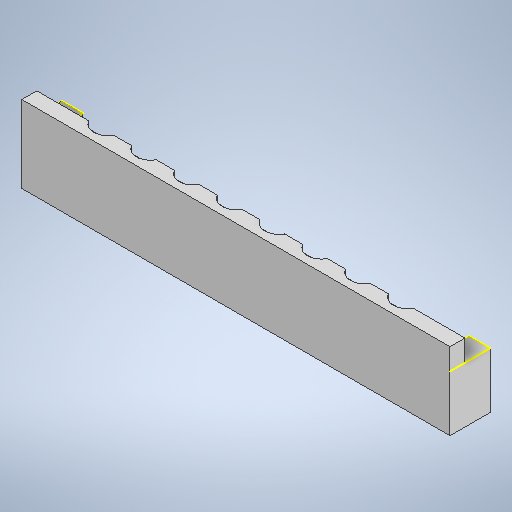
# Autodesk Inventor part: plate holder
Saved by Autodesk Inventor 2025.1 (Build 291241020, 241B)
## iProperties
Created: 2024-12-05
Part Number: plate holder
Material: Generic
Document SubType Name: Modeling
Designer: Hunter Mathis
Density: 1 g/cm^3
Appearance: Default
Author: Hunter Mathis
Autodesk Inventor part; units mm, degrees
ref_plane "YZ Plane" through (0, 0, 0) normal (1, 0, 0) x (0, 1, 0)
ref_plane "XZ Plane" through (0, 0, 0) normal (0, 1, 0) x (-1, 0, 0)
ref_plane "XY Plane" through (0, 0, 0) normal (0, 0, 1) x (1, 0, 0)
sketch "Sketch1" plane through (0, 0, 0) normal (0, 1, 0) x (-1, 0, 0)
  line L0 (63.5, -2.2225) -> (-63.5, -2.2225)
  line L1 (-63.5, -2.2225) -> (-63.5, 2.2225)
  line L2 (-63.5, 2.2225) -> (63.5, 2.2225)
  line L3 (63.5, 2.2225) -> (63.5, -2.2225)
  line L4 (63.5, -2.2225) -> (-63.5, 2.2225) construction
  line L5 (-63.5, -2.2225) -> (63.5, 2.2225) construction
  point P0 (0, 0)
  dimension "d0" = 127
  dimension "d1" = 4.445
  constraints: 12 end point, 2 midpoint, 2 parallel, 1 horizontal, 1 perpendicular
  measures "d0" distance of L1.end L2.end
  measures "d1" distance of L0.end L1.end
extrude "Extrusion1" add sketch "Sketch1" along normal blind 31.75
sketch "Sketch2" plane through (63.5, 0, -2.2225) normal (0, 0, -1) x (-1, 0, 0)
  line L0 (127, 0) -> (0, 0) projected
  line L1 (0, 0) -> (127, 0)
  line L2 (127, 0) -> (127, 25.4116)
  line L3 (127, 25.4116) -> (0, 25.4116)
  line L4 (0, 25.4116) -> (0, 0)
  point P0 (63.5, 0)
  constraints: 8 end point, 3 equal length, 1 perpendicular
extrude "Extrusion2" add sketch "Sketch2" along normal blind 7.4676
sketch "Sketch3" plane through (-63.5, 25.4116, -2.2225) normal (0, 1, 0) x (1, 0, 0)
  point P0 (63.5, -2.2225)
sketch "Sketch4" plane through (63.5, 0, -9.6901) normal (0, 0, -1) x (-1, 0, 0)
  line L0 (0, 25.4116) -> (0, 0) projected
  line L1 (6.223, 12.7058) -> (6.223, 25.4116)
  line L2 (0, 25.4116) -> (6.223, 25.4116)
  line L3 (0, 25.4116) -> (0, 12.7058)
  line L4 (0, 12.7058) -> (0, 3.1808)
  line L5 (0, 0) -> (0, 31.75) projected
  line L6 (0, 3.1808) -> (6.223, 3.1808)
  line L7 (6.223, 3.1808) -> (6.223, 12.7058)
  line L8 (0, 25.4116) -> (127, 25.4116) projected
  line L9 (127, 0) -> (127, 25.4116) projected
  line L10 (120.777, 12.7058) -> (120.777, 25.4116)
  line L11 (6.223, 25.4116) -> (120.777, 25.4116)
  line L12 (120.777, 12.7058) -> (120.777, 3.1808)
  line L13 (120.777, 3.1808) -> (127, 3.1808)
  line L14 (127, 3.1808) -> (127, 25.4116)
  line L15 (127, 0) -> (127, 31.75) projected
  line L16 (6.223, 3.1808) -> (120.777, 3.1808)
  line L17 (6.223, 3.1808) -> (6.223, 22.2308)
  line L18 (120.777, 22.2308) -> (6.223, 22.2308)
  line L19 (120.777, 22.2308) -> (120.777, 3.1808)
  line L20 (6.223, 3.1808) -> (120.777, 3.1808)
  point P0 (63.5, 0)
  point P1 (6.223, 22.2308)
  dimension "d6" = 6.223
  dimension "d7" = 9.525
  dimension "d13" = 6.223
  dimension "d14" = 19.05
  constraints: 32 end point, 5 collinear, 5 point on line, 4 perpendicular, 1 horizontal, 1 midpoint, 1 parallel, 1 vertical
  measures "d6" distance of L3.end L1.start
  measures "d7" distance of L3.end L4.end
  measures "d13" distance of L12.end L13.end
  measures "d14" distance between parallel lines of L18 L16
extrude "Extrusion3" cut sketch "Sketch4" against normal blind 4.699 contours L8 L10 L18 L1 | L18 L10 L12 L16 L7 L1
extrude "Extrusion4" add sketch "Sketch4" against normal blind 1.143 contours L18 L10 L12 L16 L7 L1
sketch "Sketch5" plane through (-63.5, 25.4116, -2.2225) normal (0, 1, 0) x (1, 0, 0)
  line L0 (127, -4.445) -> (127, 7.4676) projected
  line L1 (120.777, 7.4676) -> (120.777, 2.7686) projected
  line L2 (6.223, 2.7686) -> (6.223, 7.4676) projected
  line L3 (0, 7.4676) -> (6.223, 7.4676) projected
  line L4 (0, 0) -> (0, 7.4676) projected
  line L5 (127, 0) -> (0, 0) projected
  line L6 (127, 0) -> (127, 7.4676) projected
  line L7 (120.777, 7.4676) -> (127, 7.4676) projected
  line L8 (120.777, 2.7686) -> (6.223, 2.7686) projected
  point P0 (63.5, -2.2225)
sketch "Sketch6" plane through (-63.5, 25.4116, -2.2225) normal (0, 1, 0) x (1, 0, 0)
  point P0 (63.5, -2.2225)
sketch "Sketch7" plane through (63.5, 0, 2.2225) normal (1, 0, 0) x (0, 0, -1)
  line L0 (0, 0) -> (0, 12.7)
  line L1 (0, 0) -> (0, 31.75) projected
  line L2 (0, 12.7) -> (11.9126, 12.7)
  line L3 (10.7696, 22.2308) -> (10.7696, 3.1808) projected
  line L4 (11.9126, 25.4116) -> (11.9126, 0) projected
  line L5 (11.9126, 12.7) -> (11.9126, 0)
  line L6 (0, 0) -> (11.9126, 0) projected
  line L7 (11.9126, 0) -> (0, 0)
  point P0 (2.2225, 0)
  dimension "d26" = 12.7
  constraints: 8 end point, 2 perpendicular, 1 collinear, 1 point on line
  measures "d26" distance of L0.start L0.end
extrude "Extrusion6" cut sketch "Sketch7" against normal through all
sketch "Sketch8" plane through (63.5, 12.7, -9.6901) normal (0, -1, 0) x (1, 0, 0)
  line L0 (-127, 11.9126) -> (0, 11.9126) projected
  line L1 (0, 7.4676) -> (0, 0) projected
  line L2 (0, 11.9126) -> (0, 0)
  line L3 (0, 0) -> (-127, 0)
  line L4 (-127, 0) -> (-127, 11.9126)
  line L5 (-127, 11.9126) -> (0, 11.9126)
  point P0 (-63.5, 9.6901)
  point P1 (-127, 11.9126)
  constraints: 8 end point, 2 parallel, 1 collinear, 1 perpendicular
extrude "Extrusion7" add sketch "Sketch8" along normal blind 3.81
sketch "Sketch9" plane through (-63.5, 25.4116, -2.2225) normal (0, 1, 0) x (1, 0, 0)
  line L0 (120.777, 2.7686) -> (6.223, 2.7686) projected
  line L1 (127, 0) -> (0, 0) projected
  line L2 (120.777, 2.7686) -> (6.5121, 2.7686)
  line L3 (6.5121, 0) -> (120.777, 0)
  line L4 (120.777, 2.7686) -> (120.777, 0)
  line L5 (120.777, 0) -> (6.223, 0)
  line L6 (6.223, 0) -> (6.223, 2.7686)
  line L7 (6.223, 2.7686) -> (120.777, 2.7686)
  line L8 (120.777, 6.3246) -> (120.777, 2.7686) projected
  point P0 (63.5, -2.2225)
  point P1 (6.223, 2.7686)
  constraints: 12 end point, 2 parallel, 1 collinear, 1 horizontal, 1 perpendicular, 1 point on line
extrude "Extrusion8" cut sketch "Sketch9" against normal blind 12.7
sketch "Sketch10" plane through (63.5, 12.7, -9.6901) normal (0, 1, 0) x (1, 0, 0)
  line L0 (-6.223, 0) -> (-6.223, -1.143) projected
  line L1 (-6.223, -1.143) -> (-6.223, -4.699) projected
  line L2 (-6.223, -1.143) -> (-6.223, -2.286)
  line L3 (-6.223, -2.286) -> (-120.523, -2.286)
  line L4 (-120.523, -2.286) -> (-120.523, -1.143)
  line L5 (-120.523, -1.143) -> (-6.223, -1.143)
  point P0 (-63.5, -9.6901)
  point P1 (-6.223, -7.4676)
  constraints: 8 end point, 2 parallel, 1 perpendicular, 1 point on line
sketch "Sketch12" plane through (63.5, 31.75, -2.2225) normal (0, 0, -1) x (-1, 0, 0)
  line L0 (6.223, -6.3384) -> (6.223, -19.0384) projected
  line L1 (6.223, -6.3384) -> (6.223, -19.05)
  line L2 (6.223, -19.05) -> (120.3609, -19.05)
  line L3 (120.3609, -19.05) -> (120.3609, -6.3384)
  line L4 (120.3609, -6.3384) -> (6.223, -6.3384)
  point P0 (63.5, -31.75)
  constraints: 8 end point, 2 parallel, 1 collinear, 1 perpendicular
extrude "Extrusion11" [suppressed]
sketch "Sketch16" plane through (63.5, 0, -8.5471) normal (0, 0, 1) x (1, 0, 0)
  line L0 (-6.223, 22.2308) -> (-6.223, 12.7) projected
  line L1 (-6.223, 12.7) -> (-6.223, 22.2308)
  line L2 (-6.223, 22.2308) -> (-120.777, 22.2308)
  line L3 (-120.777, 22.2308) -> (-120.777, 12.7)
  line L4 (-120.777, 12.7) -> (-6.223, 12.7)
  point P0 (-63.5, 0)
  constraints: 8 end point, 2 parallel, 1 perpendicular, 1 vertical
extrude "Extrusion14" add sketch "Sketch16" along normal blind 2.4892
sketch "Sketch11" plane through (63.5, 8.89, -9.6901) normal (0, -1, 0) x (1, 0, 0)
  line L0 (0, 11.9126) -> (0, 7.4676) projected
  line L1 (0, 11.9126) -> (0, 7.4676)
  line L2 (0, 7.4676) -> (-6.35, 7.4676)
  line L3 (0, 11.9126) -> (-127, 11.9126) projected
  line L4 (-6.35, 11.9126) -> (-6.35, 5.5626)
  circle A0 centre (-6.35, 5.5626) radius 2.3241
  circle A1 centre (-19.05, 5.5626) radius 2.3241
  circle A2 centre (-31.75, 5.5626) radius 2.3241
  circle A3 centre (-44.45, 5.5626) radius 2.3241
  circle A4 centre (-57.15, 5.5626) radius 2.3241
  circle A5 centre (-69.85, 5.5626) radius 2.3241
  circle A6 centre (-82.55, 5.5626) radius 2.3241
  circle A7 centre (-95.25, 5.5626) radius 2.3241
  circle A8 centre (-107.95, 5.5626) radius 2.3241
  circle A9 centre (-120.65, 5.5626) radius 2.3241
  circle A10 centre (-6.35, 5.5626) radius 4.1275
  circle A11 centre (-19.05, 5.5626) radius 4.1275
  circle A12 centre (-31.75, 5.5626) radius 4.1275
  circle A13 centre (-44.45, 5.5626) radius 4.1275
  circle A14 centre (-57.15, 5.5626) radius 4.1275
  circle A15 centre (-69.85, 5.5626) radius 4.1275
  circle A16 centre (-82.55, 5.5626) radius 4.1275
  circle A17 centre (-95.25, 5.5626) radius 4.1275
  point P0 (-63.5, 9.6901)
  dimension "d38" = 6.35
  dimension "d39" = 4.6482
  dimension "d42" = 12.7
  dimension "d51" = 8.255
  dimension "d54" = 12.7
  constraints: 18 centre point, 6 end point, 2 coincident, 2 horizontal, 2 perpendicular, 1 collinear, 1 point on line, 32 other
  measures "d38" distance of L4.start L4.end
  measures "d39" diameter of A0
  measures "d42" distance of A0.centre A1.centre
  measures "d51" diameter of A10
  measures "d54" distance of A10.centre A11.centre
extrude "Extrusion10" cut sketch "Sketch11" against normal through all contours A1 | A2 | A3 | A4 | A5 | A6 | A7 | A8
sketch "Sketch13" plane through (63.5, 12.7, -9.6901) normal (0, 1, 0) x (1, 0, 0)
  circle A0 centre (-19.05, -5.5626) radius 2.3241 projected
  circle A1 centre (-19.05, -5.5626) radius 4.1275
  line L0 (-6.223, -1.143) -> (-120.777, -1.143) projected
  arc A2 (-96.5442, -3.6322) -> (-97.4077, -4.699) centre (-95.25, -5.5626) ccw projected
  arc A3 (-109.2442, -3.6322) -> (-110.1077, -4.699) centre (-107.95, -5.5626) ccw projected
  line L1 (-6.223, -3.6322) -> (-6.223, -4.699) projected
  line L2 (-120.777, -4.699) -> (-120.777, -3.6322) projected
  line L3 (-33.9077, -4.699) -> (-42.2923, -4.699) projected
  circle A4 centre (-31.75, -5.5626) radius 4.1275
  circle A5 centre (-44.45, -5.5626) radius 4.1275
  circle A6 centre (-57.15, -5.5626) radius 4.1275
  circle A7 centre (-69.85, -5.5626) radius 4.1275
  circle A8 centre (-82.55, -5.5626) radius 4.1275
  circle A9 centre (-95.25, -5.5626) radius 4.1275
  circle A10 centre (-107.95, -5.5626) radius 4.1275
  arc A11 (-45.7442, -3.6322) -> (-46.6077, -4.699) centre (-44.45, -5.5626) ccw projected
  arc A12 (-33.0442, -3.6322) -> (-33.9077, -4.699) centre (-31.75, -5.5626) ccw projected
  line L4 (-21.2077, -4.699) -> (-29.5923, -4.699) projected
  arc A13 (-20.3442, -3.6322) -> (-21.2077, -4.699) centre (-19.05, -5.5626) ccw projected
  line L5 (-6.223, -4.699) -> (-16.8923, -4.699) projected
  line L6 (-110.1077, -4.699) -> (-120.777, -4.699) projected
  line L7 (-97.4077, -4.699) -> (-105.7923, -4.699) projected
  line L8 (-84.7077, -4.699) -> (-93.0923, -4.699) projected
  arc A14 (-83.8442, -3.6322) -> (-84.7077, -4.699) centre (-82.55, -5.5626) ccw projected
  line L9 (-72.0077, -4.699) -> (-80.3923, -4.699) projected
  arc A15 (-71.1442, -3.6322) -> (-72.0077, -4.699) centre (-69.85, -5.5626) ccw projected
  line L10 (-59.3077, -4.699) -> (-67.6923, -4.699) projected
  arc A16 (-58.4442, -3.6322) -> (-59.3077, -4.699) centre (-57.15, -5.5626) ccw projected
  line L11 (-46.6077, -4.699) -> (-54.9923, -4.699) projected
  line L12 (-45.7442, -3.6322) -> (-55.8558, -3.6322) projected
  arc A17 (-54.9923, -4.699) -> (-55.8558, -3.6322) centre (-57.15, -5.5626) ccw projected
  line L13 (-33.0442, -3.6322) -> (-43.1558, -3.6322) projected
  arc A18 (-42.2923, -4.699) -> (-43.1558, -3.6322) centre (-44.45, -5.5626) ccw projected
  line L14 (-58.4442, -3.6322) -> (-68.5558, -3.6322) projected
  arc A19 (-67.6923, -4.699) -> (-68.5558, -3.6322) centre (-69.85, -5.5626) ccw projected
  line L15 (-20.3442, -3.6322) -> (-30.4558, -3.6322) projected
  arc A20 (-29.5923, -4.699) -> (-30.4558, -3.6322) centre (-31.75, -5.5626) ccw projected
  line L16 (-71.1442, -3.6322) -> (-81.2558, -3.6322) projected
  arc A21 (-80.3923, -4.699) -> (-81.2558, -3.6322) centre (-82.55, -5.5626) ccw projected
  line L17 (-6.223, -3.6322) -> (-17.7558, -3.6322) projected
  arc A22 (-16.8923, -4.699) -> (-17.7558, -3.6322) centre (-19.05, -5.5626) ccw projected
  line L18 (-83.8442, -3.6322) -> (-93.9558, -3.6322) projected
  arc A23 (-93.0923, -4.699) -> (-93.9558, -3.6322) centre (-95.25, -5.5626) ccw projected
  line L19 (-96.5442, -3.6322) -> (-106.6558, -3.6322) projected
  arc A24 (-105.7923, -4.699) -> (-106.6558, -3.6322) centre (-107.95, -5.5626) ccw projected
  line L20 (-109.2442, -3.6322) -> (-120.777, -3.6322) projected
  point P0 (-63.5, -9.6901)
  dimension "d59" = 8.255
  dimension "d62" = 12.7
  constraints: 8 centre point, 1 coincident
  measures "d59" diameter of A1
  measures "d62" distance of A1.centre A4.centre
extrude "Extrusion12" cut sketch "Sketch13" along normal blind 21.59 and the other way blind 0.889 contours A0 L5 A1 L4 | A0 L17 A1 L5 | L4 A1 L15 A0 | A0 L15 A1 L17 | A1 L17 L1 L5 | L4 A4 L15 A1 | L4 A20 L15 A4 | A4 L3 A12 L13 L15 A20 L4 | L13 A12 L3 A4 | A4 L3 A5 L13 | L13 A18 L3 A5 L11 A11 L12 | A5 L3 A18 L13 | L12 A11 L11 A5 | A5 L11 A6 L12 | L12 A17 L11 A6 L10 A16 L14 | A6 L11 A17 L12 | L14 A16 L10 A6 | A6 L10 A7 L14 | L14 A19 L10 A7 L9 A15 L16 | A7 L10 A19 L14 | L16 A15 L9 A7 | A7 L9 A8 L16 | L16 A21 L9 A8 L8 A14 L18 | A8 L9 A21 L16 | L18 A14 L8 A8 | A8 L8 A9 L18 | L18 A23 L8 A9 L7 A2 L19 | A9 L8 A23 L18 | L19 A2 L7 A9 | A9 L7 A10 L19 | L19 A24 L7 A10 L6 A3 L20 | A10 L7 A24 L19 | L20 A3 L6 A10 | A10 L6 L2 L20
body "Solid1"
